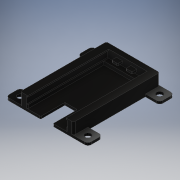
# Autodesk Inventor part: ESP32 Holder Redesign
Saved by Autodesk Inventor 2019 (Build 230136000, 136)
## iProperties
Created: 2020-01-22
Part Number: ESP32 Holder Redesign
Material: ABS Plastic
Document SubType Name: Modeling
Designer: prana
Density: 1.06 g/cm^3
Appearance: Smooth - White
Author: prana
Autodesk Inventor part; units mm, degrees
ref_plane "YZ Plane" through (0, 0, 0) normal (1, 0, 0) x (0, 1, 0)
ref_plane "XZ Plane" through (0, 0, 0) normal (0, 1, 0) x (-1, 0, 0)
ref_plane "XY Plane" through (0, 0, 0) normal (0, 0, 1) x (1, 0, 0)
sketch "Sketch1" plane through (0, 0, 0) normal (0, 1, 0) x (-1, 0, 0)
  line L0 (0, 0) -> (0, 8.89)
  line L1 (0, 8.89) -> (-8.89, 8.89)
  line L2 (-8.89, 8.89) -> (-8.89, 0)
  line L3 (-8.89, 0) -> (-44.485, 0)
  line L4 (-44.485, 0) -> (-44.485, 8.89)
  line L5 (-44.485, 8.89) -> (-53.375, 8.89)
  line L6 (-53.375, 8.89) -> (-53.375, 0)
  line L7 (-53.375, 0) -> (-53.375, -41.91)
  line L8 (-53.375, -41.91) -> (-44.485, -41.91)
  line L9 (-44.485, -41.91) -> (-44.485, -33.02)
  line L10 (-44.485, -33.02) -> (-8.89, -33.02)
  line L11 (-8.89, -33.02) -> (-8.89, -41.91)
  line L12 (-8.89, -41.91) -> (0, -41.91)
  line L13 (0, -41.91) -> (0, 0)
  circle A0 centre (-4.445, 4.445) radius 1.905
  circle A1 centre (-48.93, 4.445) radius 1.905
  circle A2 centre (-48.93, -37.465) radius 1.905
  circle A3 centre (-4.445, -37.465) radius 1.905
  dimension "d0" = 8.89
  dimension "d1" = 8.89
  dimension "d2" = 35.595
  dimension "d3" = 8.89
  dimension "d4" = 8.89
  dimension "d5" = 41.91
  dimension "d6" = 8.89
  dimension "d7" = 8.89
  dimension "d8" = 3.81
  dimension "d9" = 4.445
  dimension "d10" = 4.445
  dimension "d11" = 3.81
  dimension "d12" = 4.445
  dimension "d13" = 4.445
  dimension "d14" = 3.81
  dimension "d15" = 4.445
  dimension "d16" = 4.445
  dimension "d17" = 3.81
  dimension "d18" = 4.445
  dimension "d19" = 4.445
  constraints: 28 end point, 9 perpendicular, 4 centre point, 3 point on line, 2 vertical, 1 collinear, 1 horizontal
  measures "d0" distance of L0.start L0.end
  measures "d1" distance of L0.end L1.end
  measures "d2" distance of L2.end L3.end
  measures "d3" distance of L3.end L4.end
  measures "d4" distance of L4.end L5.end
  measures "d5" distance of L6.end L7.end
  measures "d6" distance of L7.end L8.end
  measures "d7" distance of L8.end L9.end
  measures "d8" diameter of A0
  measures "d9" distance from line of L2 A0.centre
  measures "d10" distance from line of L1 A0.centre
  measures "d11" diameter of A1
  measures "d12" distance from line of L6 A1.centre
  measures "d13" distance from line of A1.centre L5
  measures "d14" diameter of A2
  measures "d15" distance from line of A2.centre L9
  measures "d16" distance from line of L8 A2.centre
  measures "d17" diameter of A3
  measures "d18" distance from line of L13 A3.centre
  measures "d19" distance from line of L12 A3.centre
extrude "Base" add sketch "Sketch1" along normal blind 1.5
fillet "Fillet1" radius 2 8 edges at (53.375, 0.75, -41.91) (44.485, 0.75, -41.91) (53.375, 0.75, 8.89) (44.485, 0.75, 8.89) (8.89, 0.75, -41.91) (0, 0.75, -41.91) (8.89, 0.75, 8.89) (0, 0.75, 8.89)
sketch "Sketch2" plane through (0, 1.5, 0) normal (0, 1, 0) x (1, 0, 0)
  point P0 (0, 0)
sketch "Sketch3" plane through (0, 1.5, 0) normal (0, 1, 0) x (1, 0, 0)
  line L0 (53.375, -6.89) -> (53.375, 39.91) projected
  line L1 (53.375, 0) -> (0, 0)
  line L2 (0, 0) -> (0, 33.02)
  line L3 (44.485, 33.02) -> (8.89, 33.02) projected
  line L4 (0, 33.02) -> (44.485, 33.02)
  line L5 (44.485, 33.02) -> (53.375, 33.02)
  line L6 (53.375, 33.02) -> (53.375, 28.445)
  line L7 (53.375, 28.445) -> (3.175, 28.445)
  line L8 (3.175, 28.445) -> (3.175, 4.575)
  line L9 (3.175, 4.575) -> (53.375, 4.575)
  dimension "d23" = 4.575
  dimension "d24" = 3.175
  dimension "d25" = 4.575
  constraints: 16 end point, 5 point on line, 4 perpendicular, 2 horizontal
  measures "d23" distance of L5.end L6.end
  measures "d24" distance between parallel lines of L2 L8
  measures "d25" distance between parallel lines of L1 L9
extrude "bottom" add sketch "Sketch3" along normal blind 2.16 contours L1 L2 L4 L3 L5 L0 L7 L8 L9
sketch "Sketch4" plane through (0, 3.66, 0) normal (0, 1, 0) x (1, 0, 0)
  line L0 (53.375, 0) -> (53.375, 4.575) projected
  line L1 (53.375, 0) -> (0, 0)
  line L2 (53.375, 33.02) -> (0, 33.02) projected
  line L3 (0, 0) -> (0, 33.02)
  line L4 (0, 33.02) -> (53.375, 33.02)
  line L5 (53.375, 28.445) -> (53.375, 33.02) projected
  line L6 (53.375, 33.02) -> (53.375, 29.21)
  line L7 (53.375, 29.21) -> (3.175, 29.21)
  line L8 (3.175, 29.21) -> (3.175, 3.81)
  line L9 (3.175, 3.81) -> (53.375, 3.81)
  dimension "d28" = 3.81
  dimension "d29" = 3.81
  dimension "d30" = 3.175
  constraints: 14 end point, 4 perpendicular, 2 point on line, 1 collinear, 1 horizontal
  measures "d28" distance of L2.start L6.end
  measures "d29" distance between parallel lines of L9 L1
  measures "d30" distance between parallel lines of L3 L8
extrude "Extrusion3" add sketch "Sketch4" along normal blind 4.15
sketch "Sketch5" plane through (0, 7.81, 0) normal (0, 1, 0) x (1, 0, 0)
  line L0 (53.375, 0) -> (44.485, 0) projected
  line L1 (53.375, 0) -> (0, 0)
  line L2 (0, 39.91) -> (0, -6.89) projected
  line L3 (0, 33.02) -> (8.89, 33.02) projected
  line L4 (0, 33.02) -> (53.375, 33.02)
  line L5 (53.375, -6.89) -> (53.375, 39.91) projected
  line L6 (44.485, 33.02) -> (53.375, 33.02) projected
  line L7 (53.375, 33.02) -> (53.375, 28.41)
  line L8 (53.375, 4.575) -> (53.375, 28.445) projected
  line L9 (53.375, 28.41) -> (3.175, 28.41)
  line L10 (3.175, 28.445) -> (3.175, 4.575) projected
  line L11 (3.175, 28.41) -> (3.175, 4.61)
  line L12 (3.175, 4.61) -> (53.375, 4.61)
  line L13 (53.375, 3.81) -> (3.175, 3.81) projected
  line L14 (3.175, 29.21) -> (53.375, 29.21) projected
  dimension "d33" = 0.8
  dimension "d34" = 0.8
  constraints: 12 end point, 5 point on line, 2 perpendicular, 1 horizontal, 1 parallel
  measures "d33" distance between parallel lines of L13 L12
  measures "d34" distance between parallel lines of L14 L9
extrude "Extrusion4" add sketch "Sketch5" along normal blind 0.75 contours L0 L1 L2 L3 L4 L5 L9 L10 L12
sketch "Sketch6" plane through (0, 1.5, 0) normal (0, 1, 0) x (1, 0, 0)
  line L0 (53.375, 4.575) -> (53.375, 28.445) projected
  line L1 (53.375, 12.6) -> (38.375, 12.6)
  line L2 (38.375, 12.6) -> (38.375, 20.35)
  line L3 (38.375, 20.35) -> (53.375, 20.35)
  line L4 (53.375, 20.35) -> (53.375, 12.6)
  line L5 (3.175, 4.575) -> (53.375, 4.575) projected
  point P0 (0, 0)
  dimension "d37" = 7.75
  dimension "d38" = 8.025
  dimension "d39" = 15
  constraints: 8 end point, 2 parallel, 1 horizontal, 1 perpendicular, 1 point on line
  measures "d37" distance between parallel lines of L3 L1
  measures "d38" distance between parallel lines of L1 L5
  measures "d39" distance between parallel lines of L0 L2
extrude "Extrusion5" cut sketch "Sketch6" against normal blind 2
sketch "Sketch7" plane through (53.375, 1.5, -4.575) normal (0, 0, -1) x (-1, 0, 0)
  line L0 (50.2, 0) -> (0, 0) projected
  line L1 (50.2, 0) -> (47.2, 0)
  line L2 (47.2, 0) -> (47.2, 2.1371)
  line L3 (47.2, 2.1371) -> (50.2, 2.1371)
  line L4 (50.2, 2.1371) -> (50.2, 0)
  point P0 (53.375, -1.5)
  dimension "d42" = 3
  constraints: 8 end point, 2 parallel, 1 horizontal, 1 perpendicular
  measures "d42" distance between parallel lines of L2 L4
extrude "Extrusion6" add sketch "Sketch7" along normal up to next
sketch "Sketch8" plane through (3.175, 3.66, -28.445) normal (1, 0, 0) x (0, 0, -1)
  line L0 (-19.047, 2.8771) -> (-15.237, 2.8771)
  line L1 (-15.237, 2.8771) -> (-15.237, 1.6271)
  line L2 (-15.237, 1.6271) -> (-19.047, 1.6271)
  line L3 (-19.047, 1.6271) -> (-19.047, 2.8771)
  line L4 (-10.157, 2.8771) -> (-6.347, 2.8771)
  line L5 (-6.347, 2.8771) -> (-6.347, 1.6271)
  line L6 (-6.347, 1.6271) -> (-10.157, 1.6271)
  line L7 (-10.157, 1.6271) -> (-10.157, 2.8771)
  line L8 (-23.87, -0.0229) -> (0, -0.0229) projected
  line L9 (-24.635, 0) -> (-24.635, 4.15) projected
  point P0 (-28.445, -3.66)
  dimension "d45" = 1.65
  dimension "d46" = 1.65
  dimension "d47" = 5.08
  dimension "d48" = 3.81
  dimension "d49" = 3.81
  dimension "d50" = 1.25
  dimension "d51" = 1.25
  dimension "d52" = 5.588
  constraints: 16 end point, 4 parallel, 2 horizontal, 2 perpendicular
  measures "d45" distance between parallel lines of L8 L2
  measures "d46" distance between parallel lines of L8 L6
  measures "d47" distance between parallel lines of L7 L1
  measures "d48" distance between parallel lines of L5 L7
  measures "d49" distance between parallel lines of L3 L1
  measures "d50" distance between parallel lines of L6 L4
  measures "d51" distance between parallel lines of L2 L0
  measures "d52" distance between parallel lines of L9 L3
extrude "Extrusion7" add sketch "Sketch8" along normal up to surface (3 mm away)
fillet "Fillet2" radius 0.5 4 edges at (6.175, 5.9121, -13.208) (6.175, 5.9121, -9.398) (6.175, 5.9121, -18.288) (6.175, 5.9121, -22.098)
fillet "Fillet3" radius 0.5 4 edges at (38.375, 0.75, -12.6) (38.375, 0.75, -20.35) (53.375, 0.75, -12.6) (53.375, 0.75, -20.35)
fillet "Fillet4" radius 0.5 2 edges at (53.375, 2.58, -4.575) (53.375, 2.58, -28.445)
fillet "Fillet5" radius 1 4 edges at (53.375, 5.03, 0) (53.375, 5.03, -33.02) (0, 5.03, 0) (0, 5.03, -33.02)
equation "\"d53\" = d48"
body "Solid1"
